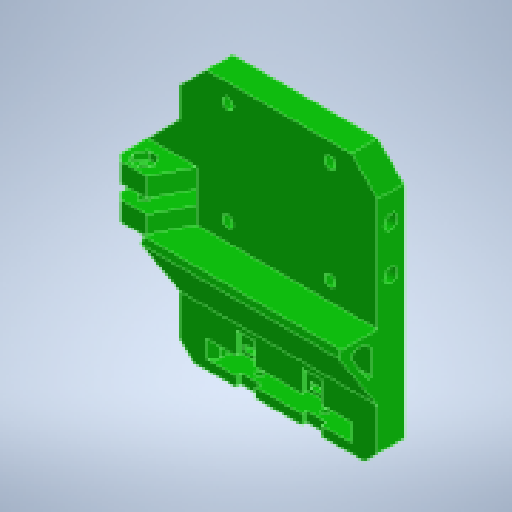
# Autodesk Inventor part: каретка_м3_без_м
Saved by Autodesk Inventor 2023.1 (Build 271208000, 208)
## iProperties
Created: 2025-12-14
Part Number: каретка_м3_без_м
Material: Латунь, мягкая, желтая, сварочная
Document SubType Name: Modeling
Designer: DELL
Density: 8.5 g/cm^3
Appearance: Темно-зеленый
Author: DELL
Autodesk Inventor part; units mm, degrees
sketch "Эскиз1" plane through (0, 0, 0) normal (0, 0, 1) x (1, 0, 0)
  line L0 (16.9838, 20.6364) -> (20.6364, 16.9838) construction
  arc A0 (16.9838, 20.6364) -> (16.3474, 20.9) centre (16.3474, 20) ccw construction
  line L1 (-16.3474, 20.9) -> (16.3474, 20.9) construction
  arc A1 (-16.3474, 20.9) -> (-16.9838, 20.6364) centre (-16.3474, 20) ccw construction
  line L2 (-20.6364, 16.9838) -> (-16.9838, 20.6364) construction
  arc A2 (-20.6364, 16.9838) -> (-20.9, 16.3474) centre (-20, 16.3474) ccw construction
  line L3 (-20.9, -16.3474) -> (-20.9, 16.3474) construction
  arc A3 (-20.9, -16.3474) -> (-20.6364, -16.9838) centre (-20, -16.3474) ccw construction
  line L4 (-16.9838, -20.6364) -> (-20.6364, -16.9838) construction
  arc A4 (-16.9838, -20.6364) -> (-16.3474, -20.9) centre (-16.3474, -20) ccw construction
  line L5 (16.3474, -20.9) -> (-16.3474, -20.9) construction
  arc A5 (16.3474, -20.9) -> (16.9838, -20.6364) centre (16.3474, -20) ccw construction
  line L6 (20.6364, -16.9838) -> (16.9838, -20.6364) construction
  arc A6 (20.6364, -16.9838) -> (20.9, -16.3474) centre (20, -16.3474) ccw construction
  line L7 (20.9, 16.3474) -> (20.9, -16.3474) construction
  arc A7 (20.9, 16.3474) -> (20.6364, 16.9838) centre (20, 16.3474) ccw construction
  circle A8 centre (15.5574, -15.5574) radius 1.45 construction
  circle A9 centre (0, 0) radius 11 construction
  circle A10 centre (-15.5574, -15.5574) radius 1.45 construction
  circle A11 centre (-15.5574, 15.5574) radius 1.45 construction
  circle A12 centre (15.5574, 15.5574) radius 1.45 construction
  circle A13 centre (0, 0) radius 11
  circle A14 centre (15.5574, 15.5574) radius 1.45
  circle A15 centre (-15.5574, 15.5574) radius 1.45
  circle A16 centre (15.5574, -15.5574) radius 1.45
  circle A17 centre (-15.5574, -15.5574) radius 1.45
  arc A18 (17.1252, 20.7778) -> (16.3474, 21.1) centre (16.3474, 20) ccw
  line L8 (17.1252, 20.7778) -> (20.7778, 17.1252)
  arc A19 (21.1, 16.3474) -> (20.7778, 17.1252) centre (20, 16.3474) ccw
  line L9 (21.1, 16.3474) -> (21.1, -16.3474)
  arc A20 (20.7778, -17.1252) -> (21.1, -16.3474) centre (20, -16.3474) ccw
  line L10 (20.7778, -17.1252) -> (17.1252, -20.7778)
  arc A21 (16.3474, -21.1) -> (17.1252, -20.7778) centre (16.3474, -20) ccw
  line L11 (16.3474, -21.1) -> (-16.3474, -21.1)
  arc A22 (-17.1252, -20.7778) -> (-16.3474, -21.1) centre (-16.3474, -20) ccw
  line L12 (-17.1252, -20.7778) -> (-20.7778, -17.1252)
  arc A23 (-21.1, -16.3474) -> (-20.7778, -17.1252) centre (-20, -16.3474) ccw
  line L13 (-21.1, -16.3474) -> (-21.1, 16.3474)
  arc A24 (-20.7778, 17.1252) -> (-21.1, 16.3474) centre (-20, 16.3474) ccw
  line L14 (-20.7778, 17.1252) -> (-17.1252, 20.7778)
  arc A25 (-16.3474, 21.1) -> (-17.1252, 20.7778) centre (-16.3474, 20) ccw
  line L15 (-16.3474, 21.1) -> (16.3474, 21.1)
  point P0 (0, 0)
  dimension "d196" = 0.2
  constraints: 16 end point, 16 point on circle, 13 centre point, 5 coincident, 5 concentric, 15 other
  measures "d196" distance between parallel lines of L1 L15
extrude "Выдавливание1" add sketch "Эскиз1" along normal blind 3 contours A14 | A15 | A16 | A17 | L8 A19 L9 A20 L10 A21 L11 A22 L12 A23 L13 A24 L14 A25 L15 A18
sketch "Эскиз2" plane through (0, 0, 3) normal (0, 0, 1) x (1, 0, 0)
  line L0 (-30, -22.9) -> (30, -22.9)
  line L1 (30, -22.9) -> (30, 21.1)
  line L2 (30, 21.1) -> (-30, 21.1)
  line L3 (-30, 21.1) -> (-30, -22.9)
  line L4 (-30, -22.9) -> (30, -22.9)
  line L5 (30, -22.9) -> (30, -57.9)
  line L6 (30, -57.9) -> (-30, -57.9)
  line L7 (-30, -57.9) -> (-30, -22.9)
  arc A0 (-16.9838, -20.6364) -> (-16.3474, -20.9) centre (-16.3474, -20) ccw
  line L8 (-16.3474, -20.9) -> (16.3474, -20.9)
  arc A1 (16.3474, -20.9) -> (16.9838, -20.6364) centre (16.3474, -20) ccw
  line L9 (20.7778, 17.1252) -> (17.1252, 20.7778) projected
  arc A2 (17.1252, 20.7778) -> (16.3474, 21.1) centre (16.3474, 20) ccw projected
  line L10 (16.3474, 21.1) -> (-16.3474, 21.1) projected
  arc A3 (-16.3474, 21.1) -> (-17.1252, 20.7778) centre (-16.3474, 20) ccw projected
  line L11 (-17.1252, 20.7778) -> (-20.7778, 17.1252) projected
  arc A4 (-20.7778, 17.1252) -> (-21.1, 16.3474) centre (-20, 16.3474) ccw projected
  line L12 (-21.1, 16.3474) -> (-21.1, -16.3474) projected
  arc A5 (-21.1, -16.3474) -> (-20.7778, -17.1252) centre (-20, -16.3474) ccw projected
  line L13 (-20.7778, -17.1252) -> (-17.1252, -20.7778) projected
  arc A6 (-17.1252, -20.7778) -> (-16.3474, -21.1) centre (-16.3474, -20) ccw projected
  line L14 (-16.3474, -21.1) -> (16.3474, -21.1) projected
  arc A7 (16.3474, -21.1) -> (17.1252, -20.7778) centre (16.3474, -20) ccw projected
  line L15 (17.1252, -20.7778) -> (20.7778, -17.1252) projected
  arc A8 (20.7778, -17.1252) -> (21.1, -16.3474) centre (20, -16.3474) ccw projected
  line L16 (21.1, -16.3474) -> (21.1, 16.3474) projected
  arc A9 (21.1, 16.3474) -> (20.7778, 17.1252) centre (20, 16.3474) ccw projected
  circle A10 centre (0, 0) radius 11 projected
  point P0 (0, 21.1)
  dimension "d4" = 60
  dimension "d5" = 60
  dimension "d6" = 35
  dimension "d232" = 44
  constraints: 16 end point, 4 parallel, 2 centre point, 2 horizontal, 2 midpoint, 2 perpendicular
  measures "d4" distance of L2.end L1.end
  measures "d5" distance of L5.end L6.end
  measures "d6" distance of L4.end L5.end
  measures "d232" distance of L0.end L1.end
extrude "Выдавливание2" add sketch "Эскиз2" against normal blind 8 contours L3 L2 A3 L11 A4 L12 A5 L13 A6 L14 A7 L15 A8 L16 A9 L9 A2 L1 L0 | L0 L5 L6 L7 | L2 A2 L9 A9 L16 A8 L15 A7 L14 A6 L13 A5 L12 A4 L11 A3 | A10
ref_plane "РабПлоскость4" through (-23, -29.9, -1) normal (0, -1, 0) x (1, 0, 0)
chamfer "Фаска1" distance 4 angle 45 2 edges at (30, -57.9, -1) (-30, -57.9, -1)
chamfer "Фаска2" distance 8 angle 45 2 edges at (30, 21.1, -1) (-30, 21.1, -1)
sketch "Эскиз25" plane through (0, 0, 3) normal (0, 0, 1) x (1, 0, 0)
  line L0 (-20, -49.6) -> (20, -49.6)
  line L1 (20, -49.6) -> (20, -54.9)
  line L2 (20, -54.9) -> (-20, -54.9)
  line L3 (-20, -54.9) -> (-20, -49.6)
  line L4 (-20, -49.6) -> (20, -54.9) construction
  line L5 (20, -49.6) -> (-20, -54.9) construction
  line L6 (-26, -57.9) -> (26, -57.9) construction
  line L7 (26, -57.9) -> (-26, -57.9) projected
  line L8 (0, -57.9) -> (0, 21.2225) construction
  point P0 (0, 0)
  point P1 (0, -52.25)
  dimension "d170" = 40
  dimension "d171" = 5.3
  dimension "d172" = 3
  constraints: 14 end point, 3 midpoint, 2 parallel, 1 horizontal, 1 perpendicular, 1 point on line
  measures "d170" distance of L1.end L2.end
  measures "d171" distance of L0.end L1.end
  measures "d172" distance between parallel lines of L6 L2
extrude "Выдавливание25" cut sketch "Эскиз25" against normal blind 8
sketch "Эскиз27" plane through (-26, -57.9, 3) normal (0, -1, 0) x (1, 0, 0)
  line L0 (0, -8) -> (0, 0) construction
  line L1 (52, 0) -> (52, -8) construction
  line L2 (0, -4) -> (52, -4) construction
  circle A0 centre (16, -4) radius 1.1
  line L3 (46, 0) -> (46, -8) construction
  line L4 (6, 0) -> (46, 0) construction
  line L5 (46, 0) -> (46, -8) construction
  line L6 (46, -8) -> (6, -8) construction
  line L7 (6, -8) -> (6, 0) construction
  line L8 (6, 0) -> (46, -8) construction
  line L9 (46, 0) -> (6, -8) construction
  circle A1 centre (36, -4) radius 1.1
  point P0 (26, -4)
  dimension "d177" = 2.2
  dimension "d178" = 10
  dimension "d179" = 2.2
  dimension "d180" = 10
  constraints: 14 end point, 5 midpoint, 2 centre point, 2 parallel, 2 point on line, 1 horizontal, 1 perpendicular
  measures "d177" diameter of A0
  measures "d178" distance from line of L7 A0.centre
  measures "d179" diameter of A1
  measures "d180" distance from line of L3 A1.centre
extrude "Выдавливание26" cut sketch "Эскиз27" against normal blind 14
sketch "Эскиз28" plane through (0, 0, 3) normal (0, 0, 1) x (1, 0, 0)
  line L0 (20, -54.9) -> (-20, -54.9) construction
  line L1 (-20, -54.9) -> (-20, -49.6) construction
  line L2 (-20, -49.6) -> (20, -49.6) construction
  line L3 (20, -49.6) -> (20, -54.9) construction
  line L4 (-26, -57.9) -> (26, -57.9) projected
  line L5 (-13, -57.9) -> (-7, -57.9)
  line L6 (-7, -57.9) -> (-7, -42.9)
  line L7 (-7, -42.9) -> (-13, -42.9)
  line L8 (-13, -42.9) -> (-13, -57.9)
  line L9 (-10, -42.9) -> (-10, -57.9) construction
  point P0 (0, 0)
  point P1 (-10, -50.4)
  point P2 (-20, -52.25)
  point P3 (-7, -55.9)
  dimension "d183" = 6
  dimension "d184" = 15
  dimension "d185" = 10
  constraints: 10 end point, 4 midpoint, 2 parallel, 1 horizontal, 1 perpendicular, 1 point on line
  measures "d183" distance of L7.end L6.end
  measures "d184" distance of L6.end L5.end
  measures "d185" horizontal distance of point (-10, -50.4) point (-20, -52.25)
extrude "Выдавливание27" cut sketch "Эскиз28" against normal blind 1.5
ref_plane "РабПлоскость8" through (0, 0, -1) normal (0, 0, -1) x (-1, 0, 0)
mirror "Зеркальное отражение4" about plane through (0, 0, 0) normal (1, 0, 0) of "Выдавливание27"
mirror "Зеркальное отражение5" about plane through (0, 0, -1) normal (0, 0, -1) of "Выдавливание27", "Зеркальное отражение4"
sketch "Эскиз29" plane through (0, 0, 1.5) normal (0, 0, 1) x (1, 0, 0)
  line L0 (-13, -42.9) -> (-7, -42.9) construction
  line L1 (-13, -49.6) -> (-13, -42.9) construction
  line L2 (7, -49.6) -> (7, -42.9) construction
  line L3 (7, -42.9) -> (13, -42.9) construction
  line L4 (-13, -42.9) -> (-7, -42.9) projected
  line L5 (-10, -42.9) -> (-10, -42.7) construction
  line L6 (-12, -46.8) -> (-8, -46.8)
  line L7 (-8, -46.8) -> (-8, -48.4)
  line L8 (-8, -48.4) -> (-12, -48.4)
  line L9 (-12, -48.4) -> (-12, -46.8)
  line L10 (-12, -46.8) -> (-8, -48.4) construction
  line L11 (-8, -46.8) -> (-12, -48.4) construction
  line L12 (-13, -49.6) -> (-7, -49.6) projected
  line L13 (7, -57.9) -> (-7, -57.9) construction
  line L14 (0, -57.9) -> (0, -38.1038) construction
  line L15 (12, -46.8) -> (8, -46.8)
  line L16 (8, -46.8) -> (8, -48.4)
  line L17 (8, -48.4) -> (12, -48.4)
  line L18 (12, -48.4) -> (12, -46.8)
  point P0 (0, 0)
  point P1 (-10, -47.6)
  dimension "d188" = 4
  dimension "d189" = 1.6
  dimension "d190" = 1.2
  constraints: 24 end point, 4 midpoint, 4 symmetric about line, 2 parallel, 2 vertical, 1 horizontal, 1 perpendicular, 1 point on line, 1 other
  measures "d188" distance of L7.end L8.end
  measures "d189" distance of L6.end L7.end
extrude "Выдавливание28" cut sketch "Эскиз29" against normal blind 10
chamfer "Фаска4" distance 2 angle 45 4 edges at (-20, -52.25, 3) (-20, -52.25, -5) (20, -52.25, 3) (20, -52.25, -5)
sketch "Эскиз30" plane through (0, 0, 3) normal (0, 0, 1) x (1, 0, 0)
  circle A0 centre (15.5, 15.45) radius 1.7 projected
  circle A1 centre (-15.5, 15.45) radius 1.7 projected
  circle A2 centre (15.5, -15.55) radius 1.7 projected
  circle A3 centre (-15.5, -15.55) radius 1.7 projected
  point P0 (0, 0)
extrude "Выдавливание29" cut sketch "Эскиз30" against normal blind 8
chamfer "Фаска7" distance 1.65 angle 45 4 edges at (-17.2, 15.45, -5) (13.8, 15.45, -5) (13.8, -15.55, -5) (-17.2, -15.55, -5)
sketch "Эскиз31" plane through (-30, -53.9, -5) normal (-1, 0, 0) x (0, 0, 1)
  line L0 (8, 75) -> (0, 75) construction
  line L1 (0, 75) -> (8, 75) construction
  line L2 (8, 75) -> (8, 32.7) construction
  line L3 (8, 32.7) -> (0, 32.7) construction
  line L4 (0, 32.7) -> (0, 75) construction
  line L5 (21, 32.7) -> (21, 12.7) construction
  line L6 (21, 12.7) -> (0, 12.7) construction
  line L7 (0, 12.7) -> (0, 32.7) construction
  line L8 (8, 67) -> (8, 0) construction
  line L9 (8, 32.7) -> (8, 12.7)
  line L10 (8, 0) -> (8, 67) projected
  line L11 (8, 12.7) -> (21, 32.7)
  line L12 (21, 32.7) -> (8, 32.7)
  line L13 (10, 30.7) -> (10, 19.4467)
  line L14 (10, 19.4467) -> (17.3146, 30.7)
  line L15 (17.3146, 30.7) -> (10, 30.7)
  point P0 (5, 53.9)
  dimension "d208" = 8
  dimension "d209" = 42.3
  dimension "d210" = 21
  dimension "d211" = 20
  dimension "d212" = 2
  constraints: 26 end point, 3 parallel, 2 perpendicular, 2 point on line, 1 horizontal, 2 other
  measures "d208" distance of L2.end L3.end
  measures "d209" distance of L1.end L2.end
  measures "d210" distance of L5.end L6.end
  measures "d211" distance of L5.start L5.end
  measures "d212" distance between parallel lines of L12 L15
extrude "Выдавливание30" add sketch "Эскиз31" against normal blind 60
chamfer "Фаска8" distance 2 angle 45 1 edges at (0, -21.2, 16)
chamfer "Фаска9" distance 2 angle 45 3 edges at (0, -23.2, 5) (0, -34.4533, 5) (0, -23.2, 12.3146)
ref_plane "РабПлоскость9" through (0, -53.9, 3) normal (1, 0, 0) x (0, 0, -1)
sketch "Эскиз37" plane through (0, 0, 3) normal (0, 0, 1) x (1, 0, 0)
  line L0 (-38, -11.8) -> (-25, -11.8) projected
  line L1 (-25, -11.8) -> (-25, -16) projected
  line L2 (-25, -16) -> (-38, -16) projected
  line L3 (-38, -23.9) -> (-38, -16) projected
  line L4 (-30, -31.9) -> (-38, -23.9) projected
  line L5 (-30, -31.9) -> (-30, -53.9) projected
  line L6 (-26, -57.9) -> (-30, -53.9) projected
  line L7 (-26, -57.9) -> (-13, -57.9) projected
  line L8 (-13, -57.9) -> (-13, -54.9) projected
  line L9 (-13, -54.9) -> (-22, -54.9) projected
  line L10 (-22, -49.6) -> (-22, -54.9) projected
  line L11 (-22, -49.6) -> (-13, -49.6) projected
  line L12 (-13, -49.6) -> (-13, -42.9) projected
  line L13 (-13, -42.9) -> (-7, -42.9) projected
  line L14 (-7, -42.9) -> (-7, -49.6) projected
  line L15 (-7, -49.6) -> (7, -49.6) projected
  line L16 (7, -49.6) -> (7, -42.9) projected
  line L17 (7, -42.9) -> (13, -42.9) projected
  line L18 (13, -42.9) -> (13, -49.6) projected
  line L19 (13, -49.6) -> (22, -49.6) projected
  line L20 (22, -54.9) -> (22, -49.6) projected
  line L21 (22, -54.9) -> (13, -54.9) projected
  line L22 (13, -54.9) -> (13, -57.9) projected
  line L23 (13, -57.9) -> (26, -57.9) projected
  line L24 (30, -53.9) -> (26, -57.9) projected
  line L25 (30, -53.9) -> (30, 13.1) projected
  line L26 (22, 21.1) -> (30, 13.1) projected
  line L27 (22, 21.1) -> (-22, 21.1) projected
  line L28 (-30, 13.1) -> (-22, 21.1) projected
  line L29 (-30, 13.1) -> (-30, 4.1) projected
  line L30 (-38, -3.9) -> (-30, 4.1) projected
  line L31 (-38, -11.8) -> (-38, -3.9) projected
  circle A0 centre (15.5574, -15.7574) radius 3.1 projected
  circle A1 centre (-15.5574, -15.7574) radius 3.1 projected
  circle A2 centre (0, -0.2) radius 13 projected
  circle A3 centre (-15.5574, 15.3574) radius 3.1 projected
  circle A4 centre (15.5574, 15.3574) radius 3.1 projected
  line L32 (-38, -3.9) -> (-40, -5.9) projected
  line L33 (-40, -5.9) -> (-40, -11.8) projected
  line L34 (-40, -11.8) -> (-38, -11.8) projected
  line L35 (-38, -11.8) -> (-38, -3.9) projected
  line L36 (-40, -21.9) -> (-38, -23.9) projected
  line L37 (-38, -23.9) -> (-38, -16) projected
  line L38 (-38, -16) -> (-40, -16) projected
  line L39 (-40, -16) -> (-40, -21.9) projected
  line L40 (-30, -21.2) -> (30, -21.2) projected
  line L41 (30, -21.2) -> (30, 13.1) projected
  line L42 (22, 21.1) -> (30, 13.1) projected
  line L43 (22, 21.1) -> (-22, 21.1) projected
  line L44 (-30, 13.1) -> (-22, 21.1) projected
  line L45 (-30, 13.1) -> (-30, -21.2) projected
  circle A5 centre (15.5, -15.55) radius 1.7 projected
  circle A6 centre (-15.5, -15.55) radius 1.7 projected
  circle A7 centre (15.5, 15.45) radius 1.7 projected
  circle A8 centre (-15.5, 15.45) radius 1.7 projected
  line L46 (-30, -41.2) -> (-30, -22.8769) projected
  line L47 (-30, -21.2) -> (-30, -22.8769) projected
  point P0 (0, 0)
  point P1 (-30, -11.8)
  point P2 (-30, -16)
extrude "Выдавливание34" add sketch "Эскиз37" against normal blind 8 contours L31 L30 L45 L0 | L34 L33 L32 L31 | L45 L47 L46 L4 L3 L2 | L3 L36 L39 L38
sketch "Эскиз38" plane through (-40, -16, 3) normal (0, 1, 0) x (1, 0, 0)
  line L0 (3.3257, 37.3) -> (1.6514, 40.2) projected
  line L1 (1.6514, 40.2) -> (3.3257, 43.1) projected
  line L2 (3.3257, 43.1) -> (6.6743, 43.1) projected
  line L3 (6.6743, 43.1) -> (8.3486, 40.2) projected
  line L4 (8.3486, 40.2) -> (6.6743, 37.3) projected
  line L5 (6.6743, 37.3) -> (3.3257, 37.3) projected
  line L6 (0, 42.2) -> (2, 44.2) projected
  line L7 (0, 42.2) -> (0, 34.2) projected
  line L8 (0, 34.2) -> (15, 34.2) projected
  line L9 (10, 44.2) -> (15, 34.2) projected
  line L10 (10, 44.2) -> (2, 44.2) projected
  line L11 (0, 0) -> (0, 34.2)
  line L12 (0, 17.1) -> (6.2707, 17.1)
  line L13 (3.3257, -3.1) -> (1.6514, -6)
  line L14 (1.6514, -6) -> (3.3257, -8.9)
  line L15 (3.3257, -8.9) -> (6.6743, -8.9)
  line L16 (6.6743, -8.9) -> (8.3486, -6)
  line L17 (8.3486, -6) -> (6.6743, -3.1)
  line L18 (6.6743, -3.1) -> (3.3257, -3.1)
  line L19 (0, -8) -> (2, -10)
  line L20 (0, -8) -> (0, 0)
  line L21 (0, 0) -> (15, 0)
  line L22 (10, -10) -> (15, 0)
  line L23 (10, -10) -> (2, -10)
  line L24 (1.6514, 40.2) -> (3.3257, 43.1) projected
  line L25 (3.3257, 37.3) -> (1.6514, 40.2) projected
  line L26 (6.6743, 37.3) -> (3.3257, 37.3) projected
  line L27 (8.3486, 40.2) -> (6.6743, 37.3) projected
  line L28 (6.6743, 43.1) -> (8.3486, 40.2) projected
  line L29 (3.3257, 43.1) -> (6.6743, 43.1) projected
  circle A0 centre (5, 40.2) radius 1.6 projected
  circle A1 centre (5, -6) radius 1.6
  point P0 (40, 3)
  point P1 (0, 17.1)
  constraints: 26 end point, 11 symmetric about line, 2 midpoint, 2 perpendicular, 1 centre point, 1 point on line, 1 other
extrude "Выдавливание35" add sketch "Эскиз38" along normal blind 10.1 and the other way blind 6 contours L18 L17 L16 L15 L14 L13 | L20 L21 L22 L23 L19
sketch "Эскиз39" plane through (-38, -5.9, 13) normal (0, 0, 1) x (1, 0, 0)
  line L0 (0, -5.9) -> (13, -5.9) projected
  line L1 (13, -5.9) -> (13, -10.1) projected
  line L2 (13, -10.1) -> (0, -10.1) projected
  line L3 (0, -18) -> (0, -10.1) projected
  line L4 (8, -26) -> (0, -18) projected
  line L5 (8, -26) -> (8, -48) projected
  line L6 (12, -52) -> (8, -48) projected
  line L7 (12, -52) -> (25, -52) projected
  line L8 (25, -52) -> (25, -49) projected
  line L9 (25, -49) -> (16, -49) projected
  line L10 (16, -43.7) -> (16, -49) projected
  line L11 (16, -43.7) -> (25, -43.7) projected
  line L12 (25, -43.7) -> (25, -37) projected
  line L13 (25, -37) -> (31, -37) projected
  line L14 (31, -37) -> (31, -43.7) projected
  line L15 (31, -43.7) -> (45, -43.7) projected
  line L16 (45, -43.7) -> (45, -37) projected
  line L17 (45, -37) -> (51, -37) projected
  line L18 (51, -37) -> (51, -43.7) projected
  line L19 (51, -43.7) -> (60, -43.7) projected
  line L20 (60, -49) -> (60, -43.7) projected
  line L21 (60, -49) -> (51, -49) projected
  line L22 (51, -49) -> (51, -52) projected
  line L23 (51, -52) -> (64, -52) projected
  line L24 (68, -48) -> (64, -52) projected
  line L25 (68, -48) -> (68, 19) projected
  line L26 (60, 27) -> (68, 19) projected
  line L27 (60, 27) -> (16, 27) projected
  line L28 (8, 19) -> (16, 27) projected
  line L29 (8, 19) -> (8, 10) projected
  line L30 (0, 2) -> (8, 10) projected
  line L31 (0, -5.9) -> (0, 2) projected
  circle A0 centre (53.5574, -9.8574) radius 3.1 projected
  circle A1 centre (22.4426, -9.8574) radius 3.1 projected
  circle A2 centre (38, 5.7) radius 13 projected
  circle A3 centre (22.4426, 21.2574) radius 3.1 projected
  circle A4 centre (53.5574, 21.2574) radius 3.1 projected
  line L32 (-2, 0) -> (-2, -16.1) projected
  line L33 (0, -16.1) -> (0, 0) projected
  line L34 (-2, 0) -> (0, 0) projected
  line L35 (-2, 0) -> (-2, -16.1) projected
  line L36 (0, -16.1) -> (-2, -16.1) projected
  line L37 (-2, -16) -> (0, -18) projected
  line L38 (0, -18) -> (0, -10.1) projected
  line L39 (0, -10.1) -> (-2, -10.1) projected
  line L40 (-2, -10.1) -> (-2, -16) projected
  line L41 (0, 2) -> (-2, 0) projected
  line L42 (-2, 0) -> (-2, -5.9) projected
  line L43 (-2, -5.9) -> (0, -5.9) projected
  line L44 (0, -5.9) -> (0, 2) projected
  point P0 (38, 5.9)
extrude "Выдавливание36" cut sketch "Эскиз39" against normal blind 20 contours L0 L1 L2 L33 | L33 L39 L32 L43
sketch "Эскиз40" plane through (-40, -5.9, 3) normal (0, 1, 0) x (1, 0, 0)
  line L0 (1.6514, 40.2) -> (3.3257, 43.1) projected
  line L1 (3.3257, 37.3) -> (1.6514, 40.2) projected
  line L2 (6.6743, 37.3) -> (3.3257, 37.3) projected
  line L3 (8.3486, 40.2) -> (6.6743, 37.3) projected
  line L4 (6.6743, 43.1) -> (8.3486, 40.2) projected
  line L5 (3.3257, 43.1) -> (6.6743, 43.1) projected
  circle A0 centre (5, 40.2) radius 1.6 projected
  line L6 (0, -8) -> (2, -10) projected
  line L7 (2, -10) -> (10, -10) projected
  line L8 (10, -10) -> (15, 0) projected
  line L9 (0, 0) -> (15, 0) projected
  line L10 (0, 0) -> (0, -8) projected
  circle A1 centre (5, -6) radius 1.6 projected
  line L11 (3.3257, 37.3) -> (1.6514, 40.2) projected
  line L12 (1.6514, 40.2) -> (3.3257, 43.1) projected
  line L13 (3.3257, 43.1) -> (6.6743, 43.1) projected
  line L14 (6.6743, 43.1) -> (8.3486, 40.2) projected
  line L15 (8.3486, 40.2) -> (6.6743, 37.3) projected
  line L16 (6.6743, 37.3) -> (3.3257, 37.3) projected
  line L17 (0, 42.2) -> (2, 44.2) projected
  line L18 (0, 42.2) -> (0, 34.2) projected
  line L19 (0, 34.2) -> (15, 34.2) projected
  line L20 (10, 44.2) -> (15, 34.2) projected
  line L21 (10, 44.2) -> (2, 44.2) projected
  line L22 (0, 34.2) -> (0, 0)
  line L23 (0, 8) -> (0, -8) projected
  line L24 (0, 17.1) -> (7.5, 17.1)
  line L25 (1.6514, -6) -> (3.3257, -8.9)
  line L26 (3.3257, -3.1) -> (1.6514, -6)
  line L27 (6.6743, -3.1) -> (3.3257, -3.1)
  line L28 (8.3486, -6) -> (6.6743, -3.1)
  line L29 (6.6743, -8.9) -> (8.3486, -6)
  line L30 (3.3257, -8.9) -> (6.6743, -8.9)
  circle A2 centre (5, -6) radius 1.6
  line L31 (3.3257, -3.1) -> (1.6514, -6)
  line L32 (1.6514, -6) -> (3.3257, -8.9)
  line L33 (3.3257, -8.9) -> (6.6743, -8.9)
  line L34 (6.6743, -8.9) -> (8.3486, -6)
  line L35 (8.3486, -6) -> (6.6743, -3.1)
  line L36 (6.6743, -3.1) -> (3.3257, -3.1)
  point P0 (40, 3)
  constraints: 28 end point, 7 symmetric about line, 1 centre point, 1 collinear, 1 horizontal, 1 midpoint, 1 other
extrude "Выдавливание37" cut sketch "Эскиз40" against normal blind 2.4 contours L26 L27 L28 L29 L30 L25
sketch "Эскиз42" plane through (30, -53.9, 3) normal (1, 0, 0) x (0, 0, -1)
  line L0 (0, 67) -> (8, 67) construction
  line L1 (4, 67) -> (4, 28.8608) construction
  circle A0 centre (4, 59) radius 2.1
  circle A1 centre (4, 45) radius 2.1
  line L2 (8, 75) -> (0, 75) projected
  point P0 (3, 53.9)
  dimension "d247" = 4.2
  dimension "d248" = 4.2
  dimension "d250" = 16
  dimension "d251" = 14
  constraints: 2 centre point, 2 end point, 2 point on line, 1 midpoint, 1 vertical
  measures "d247" diameter of A0
  measures "d248" diameter of A1
  measures "d250" distance from line of L2 A0.centre
  measures "d251" distance of A0.centre A1.centre
extrude "Выдавливание39" cut sketch "Эскиз42" against normal blind 5
